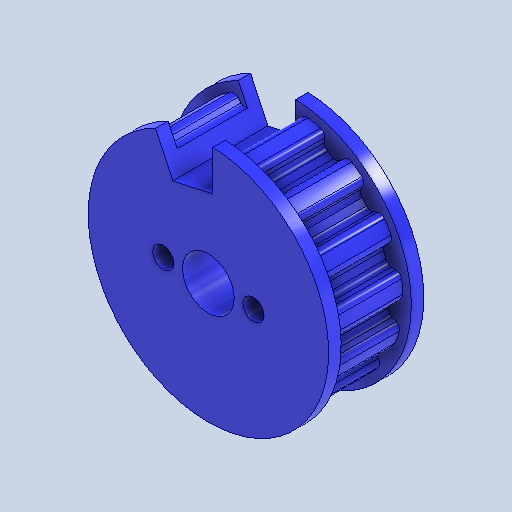
# Autodesk Inventor part: 歯付きプーリ2
Saved by Autodesk Inventor 2025.2 (Build 292293000, 293)
## iProperties
CustomPartVersion: 1
Created: 2025-01-13
Part Number: 歯付きプーリ2
Material: ABS プラスチック
Document SubType Name: Modeling
Designer: haruy
Density: 1.06 g/cm^3
Appearance: 青 - 壁塗料 - 光沢
Author: haruy
Autodesk Inventor part; units mm, degrees
ref_plane "YZ Plane" through (0, 0, 0) normal (1, 0, 0) x (0, 1, 0)
ref_plane "XZ Plane" through (0, 0, 0) normal (0, 1, 0) x (-1, 0, 0)
sketch "プーリ スケッチ" plane through (0, 0, 0) normal (0, 0, 1) x (1, 0, 0)
  circle A0 centre (0, 0) radius 22.7393 construction
  circle A1 centre (0, 0) radius 22.3583
  circle A2 centre (0, 0) radius 19.6913
  line L0 (-2.4459, 22.2241) -> (-1.524, 19.6913)
  line L1 (-1.524, 19.6913) -> (1.524, 19.6913)
  line L2 (1.524, 19.6913) -> (2.4459, 22.2241)
  line L3 (0, 0) -> (0, 22.3583) construction
  point P0 (0, 19.6913)
  dimension "d0" = 45.4785
  dimension "d1" = 0.381
  dimension "d2" = 2.667
  dimension "d3" = 40
  dimension "d4" = 3.048
  constraints: 8 end point, 3 coincident, 3 point on circle, 2 centre point, 1 horizontal, 1 midpoint, 1 point on line, 1 vertical, 1 vertical alignment, 3 other
  measures "d0" diameter of A0
  measures "d1" radial gap between concentric circles of A0 A1
  measures "d3" angle of L2 L0
  measures "d4" distance of L0.end L1.end
extrude "基本ボディ" add sketch "プーリ スケッチ" along normal mid plane 14 contours A2 | A1 L0 L1 L2 | L2 L1 L0 A1
extrude "歯" cut sketch "プーリ スケッチ" along normal through all both and the other way through all contours L2 L1 L0 A1 picked at (0, 21.4594)
fillet "Fillet" radius 1.1938 2 edges at (1.524, 19.6913, 0) (-1.524, 19.6913, 0)
fillet "Fillet" radius 1.1684 4 edges at (-2.4459, 22.2241, 3.5) (-2.4459, 22.2241, -3.5) (2.4459, 22.2241, 3.5) (2.4459, 22.2241, -3.5)
pattern_circular "Teeth" count 15 over 360 about axis through (0, 0, -10) along (0, 0, 1) of "歯", "Fillet"
sketch "スケッチ2" plane through (0, 0, 7) normal (0, 0, 1) x (1, 0, 0)
  circle A0 centre (0, 0) radius 24
  dimension "d17" = 48
  constraints: 1 centre point, 1 coincident
  measures "d17" diameter of A0
extrude "押し出し3" add sketch "スケッチ2" along normal blind 2.5
sketch "スケッチ3" plane through (0, 0, -7) normal (0, 0, -1) x (-1, 0, 0)
  circle A0 centre (0, 0) radius 5.15
  circle A1 centre (0, 0) radius 9
  circle A2 centre (-9, 0) radius 2.1
  circle A3 centre (9, 0) radius 2.1
  dimension "d21" = 18
  dimension "d20" = 10.3
  dimension "d22" = 4.2
  dimension "d25" = 360
  constraints: 3 centre point, 2 coincident, 1 horizontal alignment, 7 other
  measures "d20" diameter of A0
  measures "d22" diameter of A2
extrude "押し出し4" cut sketch "スケッチ3" against normal through all contours A0 | A1 A3 | A1 A3 | A2 A1 | A1 A2
sketch "スケッチ4" plane through (0, 0, -7) normal (0, 0, -1) x (-1, 0, 0)
  circle A0 centre (0, 0) radius 24
  arc A1 (3.4008, 22.0981) -> (2.1252, 21.3429) centre (3.2231, 20.9433) ccw projected
  arc A2 (5.8813, 21.5709) -> (3.4008, 22.0981) centre (0, 0) ccw projected
  line L0 (3.4008, 22.0981) -> (5.8813, 21.5709)
  circle A3 centre (0, 0) radius 22.3583
  line L1 (3.0166, 22.2166) -> (7.6378, 21.2343)
  line L2 (0.736, 22.7013) -> (8.5611, 21.038)
  line L3 (8.5611, 21.038) -> (7.1058, 14.191)
  line L4 (7.1058, 14.191) -> (-0.7194, 15.8543)
  line L5 (-0.7194, 15.8543) -> (0.736, 22.7013)
  line L6 (-0.7194, 15.8543) -> (-0.8968, 23.9832)
  circle A4 centre (0, 0) radius 24 projected
  line L7 (0, 0) -> (4.6485, 21.8697)
  line L8 (7.1058, 14.191) -> (10.5741, 21.545)
  point P0 (10.5741, 21.545)
  point P1 (10.5741, 21.545)
  dimension "d29" = 48
  dimension "d30" = 0
  dimension "d31" = 7
  dimension "d32" = 8
  dimension "d33" = 4
  dimension "d34" = 13.25
  constraints: 18 end point, 3 parallel, 3 point on circle, 2 centre point, 2 coincident, 2 perpendicular, 2 point on line, 1 symmetric about line, 1 tangent, 2 other
  measures "d29" diameter of A0
  measures "d30" distance from line of point (4.649, 21.87) L1
  measures "d31" distance of L2.end L3.end
  measures "d32" distance between parallel lines of L3 L5
  measures "d33" distance from line of L7.end L5
extrude "押し出し5" cut sketch "スケッチ4" against normal through all contours L8 A3 L3 L2 L1 L5 L6 A0 | L8 L3 A3 | A3 L5 L6 | L3 L4 L7 L0 A3 | A3 A2 L1 L2 L3 | L5 L2 L1 A2 A3 | A3 L0 L7 L4 L5 | L0 L7 A2 | A2 L7 L0
sketch "スケッチ5" plane through (0, 0, 9.5) normal (0, 0, 1) x (1, 0, 0)
  line L0 (-7.1058, 14.191) -> (-10.5741, 21.545) projected
  arc A0 (-10.5741, 21.545) -> (0.8968, 23.9832) centre (0, 0) ccw projected
  line L1 (0.8968, 23.9832) -> (0.7194, 15.8543) projected
  line L2 (0.7194, 15.8543) -> (-7.1058, 14.191) projected
  circle A1 centre (-9, 0) radius 2.1 projected
  circle A2 centre (9, 0) radius 2.1 projected
  circle A3 centre (0, 0) radius 5.15 projected
ref_plane "作業平面1" through (0, 0, 0) normal (0, 0, -1) x (-1, 0, 0)
mirror "ミラー1" about plane through (0, 0, 0) normal (0, 0, -1) of "押し出し3", "押し出し5", "押し出し4"
equation "\"d1\" = da_a"
equation "\"d2\" = da_hg"
equation "\"d3\" = 2 * da_fi"
equation "\"d4\" = da_bw"
equation "\"d5\" = da_bf"
equation "\"d7\" = da_bf"
equation "\"d9\" = da_rb"
equation "\"d10\" = da_rt"
equation "\"da_pb\" = 9.525"
equation "\"da_fi\" = 20deg"
equation "\"da_hg\" = 2.667"
equation "\"da_bw\" = 3.048"
equation "\"da_rb\" = 1.1938"
equation "\"da_rt\" = 1.1684"
equation "\"da_a\" = 0.381"
equation "\"da_bf\" = 14"
equation "\"da_wf\" = 1.27"
equation "\"da_hf\" = 1.651"
body "Solid1"
